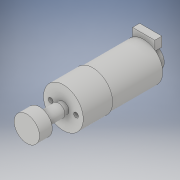
# Autodesk Inventor part: Motor_Place_Holder
Saved by Autodesk Inventor 2018.2 (Build 222227000, 227)
## iProperties
Created: 2018-08-09
Part Number: Motor_Place_Holder
Material: Generic
Document SubType Name: Modeling
Designer: mateu
Density: 1 g/cm^3
Appearance: Default
Author: mateu
Autodesk Inventor part; units mm, degrees
ref_plane "YZ Plane" through (0, 0, 0) normal (1, 0, 0) x (0, 1, 0)
ref_plane "XZ Plane" through (0, 0, 0) normal (0, 1, 0) x (-1, 0, 0)
ref_plane "XY Plane" through (0, 0, 0) normal (0, 0, 1) x (1, 0, 0)
sketch "Sketch1" plane through (0, 0, 0) normal (0, 0, 1) x (1, 0, 0)
  circle A0 centre (0, 0) radius 12
  dimension "d0" = 24
  constraints: 1 centre point, 1 coincident
  measures "d0" diameter of A0
extrude "Extrusion1" add sketch "Sketch1" along normal blind 32
sketch "Sketch2" plane through (0, 0, 32) normal (0, 0, 1) x (1, 0, 0)
  circle A0 centre (0, 0) radius 12.5
  dimension "d3" = 25
  constraints: 1 centre point, 1 coincident
  measures "d3" diameter of A0
sketch "Sketch3" plane through (0, 0, 32) normal (0, 0, 1) x (1, 0, 0)
  point P0 (0, 0)
extrude "Extrusion2" add sketch "Sketch2" along normal blind 18.5
sketch "Sketch4" plane through (0, 0, 50.5) normal (0, 0, 1) x (1, 0, 0)
  circle A0 centre (0, 0) radius 3.5
  dimension "d6" = 7
  constraints: 1 centre point, 1 coincident
  measures "d6" diameter of A0
extrude "Extrusion3" add sketch "Sketch4" along normal blind 3
sketch "Sketch7" plane through (0, 0, 0) normal (0, 0, -1) x (-1, 0, 0)
  circle A0 centre (0, 0) radius 7
  dimension "d15" = 14
  constraints: 1 centre point, 1 coincident
  measures "d15" diameter of A0
extrude "Extrusion6" add sketch "Sketch7" along normal blind 6
sketch "Sketch8" plane through (0, 0, 0) normal (0, 0, -1) x (-1, 0, 0)
  circle A0 centre (0, 0) radius 12 projected
  line L0 (0, 9) -> (7, 9)
  line L1 (7, 9) -> (7, 15)
  line L2 (7, 15) -> (-7, 15)
  line L3 (-7, 15) -> (-7, 9)
  line L4 (-7, 9) -> (0, 9)
  dimension "d20" = 7
  dimension "d21" = 14
  constraints: 10 end point, 3 perpendicular, 1 collinear, 1 point on line
  measures "d20" distance of L0.start L0.end
  measures "d21" distance of L1.end L2.end
extrude "Extrusion7" add sketch "Sketch8" along normal blind 4.5 contours L1 L0 L4 L3 A0 | A0 L3 L2 L1 picked at (-3.7936, 9.7239)
sketch "Sketch9" plane through (0, 0, 50.5) normal (0, 0, 1) x (1, 0, 0)
  circle A0 centre (-8, 0) radius 1.5
  circle A1 centre (8, 0) radius 1.5
  point P0 (0, 0)
  dimension "d24" = 3
  dimension "d25" = 8
  dimension "d26" = 3
  dimension "d27" = 8
  constraints: 2 centre point
  measures "d24" diameter of A0
  measures "d25" distance of point (0, 0) A0.centre
  measures "d26" diameter of A1
  measures "d27" distance of point (0, 0) A1.centre
extrude "Extrusion8" cut sketch "Sketch9" against normal blind 5
sketch "Sketch10" plane through (0, 0, 53.5) normal (0, 0, 1) x (1, 0, 0)
  circle A0 centre (0, 0) radius 4
  dimension "d30" = 8
  constraints: 1 centre point, 1 coincident
  measures "d30" diameter of A0
extrude "Extrusion9" add sketch "Sketch10" along normal blind 12
sketch "Sketch11" plane through (0, 0, 65.5) normal (0, 0, 1) x (1, 0, 0)
  circle A0 centre (0, 0) radius 7 projected
  circle A1 centre (0, 0) radius 8
  dimension "d33" = 16
  constraints: 1 centre point, 1 coincident
  measures "d33" diameter of A1
extrude "Extrusion10" add sketch "Sketch11" along normal blind 8 contours A0 | A1
body "Solid1"
